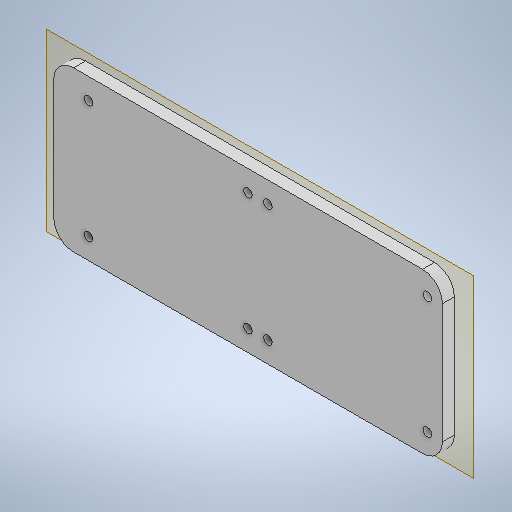
# Autodesk Inventor part: led 7 seg v3_bottom
Saved by Autodesk Inventor 2026 (Build 300175000, 175)
## iProperties
Created: 2025-07-04
Part Number: led 7 seg v3_bottom
Material: Generic
Document SubType Name: Modeling
Designer: Korobeynikov
Density: 1 g/cm^3
Appearance: Default
Author: Korobeynikov
Autodesk Inventor part; units mm, degrees
ref_plane "YZ Plane" through (0, 0, 0) normal (1, 0, 0) x (0, 1, 0)
ref_plane "XZ Plane" through (0, 0, 0) normal (0, 1, 0) x (-1, 0, 0)
ref_plane "XY Plane" through (0, 0, 0) normal (0, 0, 1) x (1, 0, 0)
ref_plane "Work Plane1" through (0, 0, 0) normal (0, 0, 1) x (1, 0, 0)
sketch "Sketch1" plane through (0, 0, 0) normal (0, 0, 1) x (1, 0, 0)
  arc A0 (87.5, -38) -> (95.5, -30) centre (87.5, -30) ccw projected
  line L0 (87.5, -38) -> (-87.5, -38) projected
  arc A1 (-95.5, -30) -> (-87.5, -38) centre (-87.5, -30) ccw projected
  line L1 (-95.5, -30) -> (-95.5, 30) projected
  arc A2 (-87.5, 38) -> (-95.5, 30) centre (-87.5, 30) ccw projected
  line L2 (-87.5, 38) -> (87.5, 38) projected
  arc A3 (95.5, 30) -> (87.5, 38) centre (87.5, 30) ccw projected
  line L3 (95.5, 30) -> (95.5, -30) projected
  line L4 (-87.5, -40) -> (87.5, -40) projected
  arc A4 (87.5, -40) -> (97.5, -30) centre (87.5, -30) ccw projected
  line L5 (97.5, -30) -> (97.5, 30) projected
  arc A5 (97.5, 30) -> (87.5, 40) centre (87.5, 30) ccw projected
  line L6 (87.5, 40) -> (-87.5, 40) projected
  arc A6 (-87.5, 40) -> (-97.5, 30) centre (-87.5, 30) ccw projected
  line L7 (-97.5, 30) -> (-97.5, -30) projected
  arc A7 (-97.5, -30) -> (-87.5, -40) centre (-87.5, -30) ccw projected
  point P0 (0, 0)
extrude "Extrusion1" add sketch "Sketch1" along normal blind 4
sketch "Sketch2" plane through (0, 0, 4) normal (0, 0, 1) x (1, 0, 0)
  arc A0 (87.5, -40) -> (97.5, -30) centre (87.5, -30) ccw projected
  line L0 (97.5, -30) -> (97.5, 30) projected
  arc A1 (97.5, 30) -> (87.5, 40) centre (87.5, 30) ccw projected
  line L1 (87.5, 40) -> (-87.5, 40) projected
  arc A2 (-87.5, 40) -> (-97.5, 30) centre (-87.5, 30) ccw projected
  line L2 (-97.5, 30) -> (-97.5, -30) projected
  arc A3 (-97.5, -30) -> (-87.5, -40) centre (-87.5, -30) ccw projected
  line L3 (-87.5, -40) -> (87.5, -40) projected
  line L4 (-95.5, -30) -> (-95.5, 30) projected
  arc A4 (-87.5, 38) -> (-95.5, 30) centre (-87.5, 30) ccw projected
  line L5 (-87.5, 38) -> (87.5, 38) projected
  arc A5 (95.5, 30) -> (87.5, 38) centre (87.5, 30) ccw projected
  line L6 (95.5, 30) -> (95.5, -30) projected
  arc A6 (87.5, -38) -> (95.5, -30) centre (87.5, -30) ccw projected
  line L7 (87.5, -38) -> (-87.5, -38) projected
  arc A7 (-95.5, -30) -> (-87.5, -38) centre (-87.5, -30) ccw projected
  circle A8 centre (-80, -29.5) radius 2.15 projected
  circle A9 centre (0, -29.5) radius 2.15 projected
  circle A10 centre (-80, 29.5) radius 2.15 projected
  circle A11 centre (0, 29.5) radius 2.15 projected
  circle A12 centre (10, 29.5) radius 2.15 projected
  circle A13 centre (10, -29.5) radius 2.15 projected
  circle A14 centre (90, -29.5) radius 2.15 projected
  circle A15 centre (90, 29.5) radius 2.15 projected
  circle A16 centre (-80, 29.5) radius 1.75
  circle A17 centre (-80, -29.5) radius 1.75
  circle A18 centre (0, -29.5) radius 1.75
  circle A19 centre (10, -29.5) radius 1.75
  circle A20 centre (0, 29.5) radius 1.75
  circle A21 centre (10, 29.5) radius 1.75
  circle A22 centre (90, 29.5) radius 1.75
  circle A23 centre (90, -29.5) radius 1.75
  point P0 (0, 0)
  dimension "d2" = 3.5
  dimension "d3" = 3.5
  dimension "d4" = 3.5
  dimension "d5" = 3.5
  dimension "d6" = 3.5
  dimension "d7" = 3.5
  dimension "d8" = 3.5
  dimension "d9" = 3.5
  constraints: 8 centre point, 8 coincident
  measures "d2" diameter of A16
  measures "d3" diameter of A17
  measures "d4" diameter of A18
  measures "d5" diameter of A19
  measures "d6" diameter of A20
  measures "d7" diameter of A21
  measures "d8" diameter of A22
  measures "d9" diameter of A23
extrude "Extrusion2" add sketch "Sketch2" along normal blind 2 contours L3 A3 L2 A2 L1 A1 L0 A0 | L4 A4 L5 A5 L6 A6 L7 A7
sketch "Sketch3" plane through (0, 0, 4) normal (0, 0, -1) x (-1, 0, 0)
  circle A0 centre (80, 29.5) radius 2.15 projected
  circle A1 centre (80, 29.5) radius 4.5
  circle A2 centre (80, -29.5) radius 2.15 projected
  circle A3 centre (80, -29.5) radius 4.5
  circle A4 centre (0, 29.5) radius 2.15 projected
  circle A5 centre (0, 29.5) radius 4.5
  circle A6 centre (0, -29.5) radius 2.15 projected
  circle A7 centre (0, -29.5) radius 4.5
  circle A8 centre (-10, 29.5) radius 2.15 projected
  circle A9 centre (-10, 29.5) radius 4.5
  circle A10 centre (-10, -29.5) radius 2.15 projected
  circle A11 centre (-10, -29.5) radius 4.5
  circle A12 centre (-90, 29.5) radius 2.15 projected
  circle A13 centre (-90, 29.5) radius 4.5
  circle A14 centre (-90, -29.5) radius 2.15 projected
  circle A15 centre (-90, -29.5) radius 4.5
  point P0 (0, 0)
  dimension "d17" = 9
  constraints: 8 centre point, 8 coincident, 7 equal radius
  measures "d17" diameter of A11
extrude "Extrusion3" add sketch "Sketch3" along normal blind 2
sketch "Sketch4" plane through (0, 0, 4) normal (0, 0, -1) x (-1, 0, 0)
  line L0 (75, 36) -> (-75, 36)
  line L1 (-75, 36) -> (-75, 38)
  line L2 (-75, 38) -> (75, 38)
  line L3 (75, 38) -> (75, 36)
  line L4 (87.5, 38) -> (-87.5, 38) projected
  line L5 (-75, -36) -> (75, -36)
  line L6 (75, -38) -> (-75, -38)
  line L7 (75, -36) -> (75, -38)
  line L8 (-75, -38) -> (-75, -36)
  line L9 (-95.5, 20) -> (-93.5, 20)
  line L10 (-93.5, 20) -> (-93.5, -20)
  line L11 (-93.5, -20) -> (-95.5, -20)
  line L12 (-95.5, -20) -> (-95.5, 20)
  line L13 (-95.5, 30) -> (-95.5, -30) projected
  line L14 (93.5, 20) -> (95.5, 20)
  line L15 (95.5, 20) -> (95.5, -20)
  line L16 (95.5, -20) -> (93.5, -20)
  line L17 (93.5, -20) -> (93.5, 20)
  line L18 (95.5, -30) -> (95.5, 30) projected
  point P0 (0, 0)
  point P1 (0, 38)
  point P2 (0, -38)
  point P3 (-95.5, 0)
  point P4 (95.5, 0)
  dimension "d22" = 2
  dimension "d23" = 150
  dimension "d26" = 360
  dimension "d30" = 2
  dimension "d31" = 40
  constraints: 32 end point, 6 midpoint, 6 parallel, 3 horizontal, 3 perpendicular, 2 equal length, 19 other
  measures "d22" distance between parallel lines of L2 L0
  measures "d23" distance of L0.start L0.end
  measures "d30" distance of L9.start L9.end
  measures "d31" distance of L9.end L10.end
extrude "Extrusion4" add sketch "Sketch4" along normal blind 6 contours L0 L1 L2 L3 | L5 L7 L6 L8 | L14 L15 L16 L17
sketch "Sketch7" plane through (0, 0, -2) normal (0, 0, -1) x (-1, 0, 0)
  line L0 (93.5, -20) -> (93.5, 20) projected
  line L1 (97.5, 30) -> (97.5, -30) projected
  line L2 (93.5, 2.5) -> (97.5, 2.5)
  line L3 (97.5, 2.5) -> (97.5, -2.5)
  line L4 (97.5, -2.5) -> (93.5, -2.5)
  line L5 (93.5, -2.5) -> (93.5, 2.5)
  point P0 (0, 0)
  point P1 (93.5, 0)
  dimension "d38" = 5
  constraints: 8 end point, 2 midpoint, 2 parallel, 2 point on line, 1 horizontal, 1 perpendicular
  measures "d38" distance between parallel lines of L4 L2
extrude "Extrusion7" cut sketch "Sketch7" against normal blind 4
body "Solid1"
